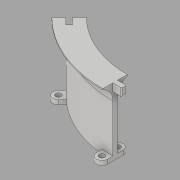
# Autodesk Inventor part: UnderTrack
Saved by Autodesk Inventor 2017 (Build 210142000, 142)
## iProperties
Created: 2019-05-24
Part Number: UnderTrack
Material: Generic
Document SubType Name: Modeling
Designer: Joe Sedutto
Density: 1 g/cm^3
Appearance: Default
Author: Joe Sedutto
Autodesk Inventor part; units mm, degrees
ref_plane "YZ Plane" through (0, 0, 0) normal (1, 0, 0) x (0, 1, 0)
ref_plane "XZ Plane" through (0, 0, 0) normal (0, 1, 0) x (-1, 0, 0)
ref_plane "XY Plane" through (0, 0, 0) normal (0, 0, 1) x (1, 0, 0)
sketch "Sketch1" plane through (0, 0, 0) normal (0, 1, 0) x (-1, 0, 0)
  line L0 (0, 0) -> (0, -27.94)
  arc A0 (79.9243, -61.0457) -> (0, -27.94) centre (0, -140.97) ccw
  arc A1 (99.6808, -41.2892) -> (0, 0) centre (0, -140.97) ccw
  line L1 (99.6808, -41.2892) -> (79.9243, -61.0457)
  line L2 (0, -27.94) -> (0, -140.97) construction
  line L3 (0, -140.97) -> (79.9243, -61.0457) construction
  point P0 (0, -13.97)
  dimension "d0" = 27.94
  dimension "d1" = 45
  dimension "d2" = 127
  constraints: 8 end point, 4 point on circle, 2 centre point, 1 coincident, 1 collinear, 1 equal length, 1 midpoint, 1 vertical
  measures "d0" distance of L0.start L0.end
  measures "d1" angle of L1 L0
  measures "d2" distance of A0.centre point (0, -13.97)
extrude "Extrusion1" add sketch "Sketch1" along normal blind 1.27
sketch "Sketch2" plane through (0, 0, 0) normal (0, -1, 0) x (1, 0, 0)
  line L0 (0, 0) -> (0, -27.94) projected
  arc A0 (0, 0) -> (-99.6808, -41.2892) centre (0, -140.97) ccw projected
  line L1 (-79.9243, -61.0457) -> (-99.6808, -41.2892) projected
  arc A1 (0, -27.94) -> (-79.9243, -61.0457) centre (0, -140.97) ccw projected
  arc A2 (0, -11.43) -> (-91.5986, -49.3714) centre (-0.0024, -140.9641) ccw
  arc A3 (0, -16.51) -> (-88.0065, -52.9635) centre (-0.0024, -140.9641) ccw
  line L2 (0, -11.43) -> (0, -16.51)
  line L3 (-91.5986, -49.3714) -> (-88.0065, -52.9635)
  line L4 (0, 0) -> (0, -27.94) projected
  line L5 (0, 0) -> (0, -27.94) projected
  point P0 (-89.8026, -51.1674)
  dimension "d5" = 5.08
  dimension "d6" = 11.43
  dimension "d7" = 11.43
  constraints: 4 end point, 4 point on circle, 2 centre point, 2 collinear, 1 coincident, 1 equal length, 1 midpoint, 1 vertical
  measures "d5" distance of L2.start L2.end
  measures "d6" distance of L4.start L2.start
  measures "d7" distance of L1.end L3.start
extrude "Extrusion2" add sketch "Sketch2" along normal blind 76.2 contours L0 A3 L1 A2
fillet "Fillet1" radius 17.78 2 edges at (-49.573, 0, -21.2902) (-47.629, 0, -25.9835)
sketch "Sketch3" plane through (0, -76.2, 0) normal (0, -1, 0) x (1, 0, 0)
  circle A0 centre (-6.35, -23.0307) radius 3.175
  circle A1 centre (-6.35, -23.0307) radius 6.35
  circle A2 centre (-6.35, -5.2283) radius 3.175
  circle A3 centre (-6.35, -5.2283) radius 6.35
  line L0 (-12.7, -5.2283) -> (-12.7, -23.0307)
  line L1 (0, -5.2283) -> (0, -23.0307)
  arc A4 (0, -11.43) -> (-91.5986, -49.3714) centre (-0.0024, -140.9641) ccw projected
  arc A5 (0, -16.51) -> (-88.0065, -52.9635) centre (-0.0024, -140.9641) ccw projected
  line L2 (0, -16.51) -> (0, -11.43) projected
  circle A6 centre (-91.4937, -40.496) radius 3.175
  circle A7 centre (-91.4937, -40.496) radius 6.35
  circle A8 centre (-78.9056, -53.0842) radius 3.175
  circle A9 centre (-78.9056, -53.0842) radius 6.35
  line L3 (-95.9838, -44.9862) -> (-83.3957, -57.5743)
  line L4 (-87.0036, -36.0059) -> (-74.4154, -48.5941)
  line L5 (-91.5986, -49.3714) -> (-88.0065, -52.9635) projected
  point P0 (0, 0)
  dimension "d11" = 6.35
  dimension "d12" = 12.7
  dimension "d13" = 6.35
  dimension "d14" = 12.7
  constraints: 12 tangent, 8 centre point, 8 end point, 8 point on circle, 4 coincident, 4 equal radius, 2 collinear
  measures "d11" diameter of A0
  measures "d12" diameter of A1
  measures "d13" diameter of A2
  measures "d14" diameter of A3
extrude "Extrusion3" add sketch "Sketch3" against normal blind 5.08
sketch "Sketch4" plane through (0, 1.27, 0) normal (1, 0, 0) x (0, 0, -1)
  line L0 (0, 0) -> (27.94, 0) projected
  line L1 (11.43, 0) -> (16.51, 0)
  line L2 (16.51, 0) -> (16.51, -8.89)
  line L3 (16.51, -8.89) -> (11.43, -8.89)
  line L4 (11.43, -8.89) -> (11.43, 0)
  point P0 (0, -1.27)
  dimension "d17" = 11.43
  dimension "d18" = 11.43
  dimension "d19" = 8.89
  constraints: 8 end point, 2 parallel, 1 horizontal, 1 perpendicular, 1 point on line
  measures "d17" distance from line of L4 L0.start
  measures "d18" distance from line of L2 L0.end
  measures "d19" distance between parallel lines of L0 L3
extrude "Extrusion4" add sketch "Sketch4" along normal blind 10.16
sketch "Sketch5" plane through (-88.0065, -71.12, -52.9635) normal (-0.7071068, 0, -0.7071068) x (-0.7071068, 0, 0.7071068)
  line L0 (16.51, 72.39) -> (-24.7792, 72.39) projected
  line L1 (-0.127, 72.39) -> (5.207, 72.39)
  line L2 (5.207, 72.39) -> (5.207, 63.5)
  line L3 (5.207, 63.5) -> (-0.127, 63.5)
  line L4 (-0.127, 63.5) -> (-0.127, 72.39)
  line L5 (-11.43, 72.39) -> (16.51, 72.39) projected
  point P0 (-24.7792, 71.12)
  dimension "d22" = 11.303
  dimension "d23" = 11.303
  dimension "d24" = 8.89
  constraints: 8 end point, 2 parallel, 1 horizontal, 1 perpendicular, 1 point on line
  measures "d22" distance from line of L4 L5.start
  measures "d23" distance from line of L0.start L2
  measures "d24" distance of L1.end L2.end
extrude "Extrusion5" cut sketch "Sketch5" against normal blind 10.16
fillet "Fillet2" radius 1.27 3 edges at (10.16, -7.62, -13.97) (10.16, -3.175, -11.43) (10.16, -3.175, -16.51)
body "Solid1"
